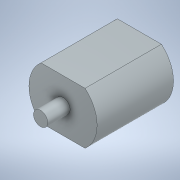
# Autodesk Inventor part: dc_motor
Saved by Autodesk Inventor 2020 (Build 240168000, 168)
## iProperties
Created: 2021-03-06
Part Number: dc_motor
Material: Generic
Document SubType Name: Modeling
Designer: Harry
Density: 1 g/cm^3
Appearance: Zinc
Author: Harry
Autodesk Inventor part; units mm, degrees
ref_plane "YZ Plane" through (0, 0, 0) normal (1, 0, 0) x (0, 1, 0)
ref_plane "XZ Plane" through (0, 0, 0) normal (0, 1, 0) x (-1, 0, 0)
ref_plane "XY Plane" through (0, 0, 0) normal (0, 0, 1) x (1, 0, 0)
sketch "Sketch1" plane through (0, 0, 0) normal (0, 0, 1) x (1, 0, 0)
  line L0 (7.7639, -9.15) -> (-7.7639, -9.15)
  line L1 (-7.7639, -9.15) -> (-7.7639, 9.15) construction
  line L2 (-7.7639, 9.15) -> (7.7639, 9.15)
  line L3 (7.7639, -9.15) -> (-7.7639, 9.15) construction
  line L4 (-7.7639, -9.15) -> (7.7639, 9.15) construction
  arc A0 (-7.7639, 9.15) -> (-7.7639, -9.15) centre (0, 0) ccw
  arc A1 (7.7639, -9.15) -> (7.7639, 9.15) centre (0, 0) ccw
  dimension "d8" = 18.3
  constraints: 10 end point, 4 point on circle, 2 centre point, 2 midpoint, 1 horizontal, 1 parallel, 1 perpendicular
  measures "d8" distance of L0.end L1.end
extrude "Extrusion1" add sketch "Sketch1" along normal blind 26.9
sketch "Sketch2" plane through (0, 0, 26.9) normal (0, 0, 1) x (1, 0, 0)
  circle A0 centre (0, 0) radius 2.5
  dimension "d4" = 5
  constraints: 1 centre point, 1 coincident
  measures "d4" diameter of A0
extrude "Extrusion2" add sketch "Sketch2" along normal blind 7.9
body "Solid1"
